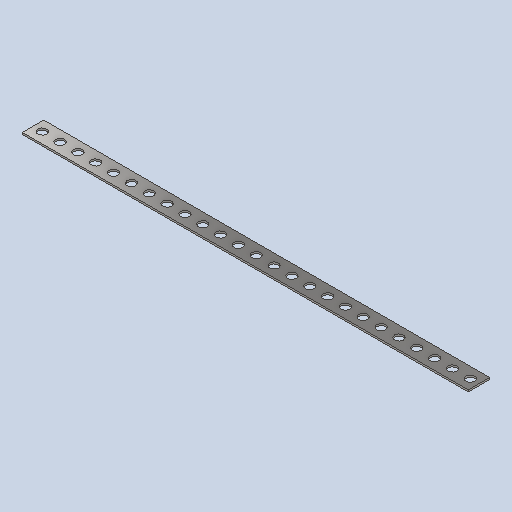
# Autodesk Inventor part: aste
Saved by Autodesk Inventor 2023 (Build 270158000, 158)
## iProperties
Created: 2023-08-07
Part Number: aste
Material: Aço, carbono
Document SubType Name: Modeling
Designer: azeve
Density: 7.85 g/cm^3
Appearance: Semipolido
Author: azeve
Autodesk Inventor part; units mm, degrees
ref_plane "YZ Plane" through (0, 0, 0) normal (1, 0, 0) x (0, 1, 0)
ref_plane "XZ Plane" through (0, 0, 0) normal (0, 1, 0) x (-1, 0, 0)
ref_plane "XY Plane" through (0, 0, 0) normal (0, 0, 1) x (1, 0, 0)
sketch "Esboço1" plane through (0, 0, 0) normal (0, 1, 0) x (-1, 0, 0)
  line L0 (0, 0) -> (250, 0)
  line L1 (250, 0) -> (250, 12)
  line L2 (250, 12) -> (0, 12)
  line L3 (0, 12) -> (0, 0)
  circle A0 centre (4.8421, 6) radius 2.5
  circle A1 centre (14.8421, 6) radius 2.5
  circle A2 centre (24.8421, 6) radius 2.5
  circle A3 centre (34.8421, 6) radius 2.5
  circle A4 centre (44.8421, 6) radius 2.5
  circle A5 centre (54.8421, 6) radius 2.5
  circle A6 centre (64.8421, 6) radius 2.5
  circle A7 centre (74.8421, 6) radius 2.5
  circle A8 centre (84.8421, 6) radius 2.5
  circle A9 centre (94.8421, 6) radius 2.5
  circle A10 centre (104.8421, 6) radius 2.5
  circle A11 centre (114.8421, 6) radius 2.5
  circle A12 centre (124.8421, 6) radius 2.5
  circle A13 centre (134.8421, 6) radius 2.5
  circle A14 centre (144.8421, 6) radius 2.5
  circle A15 centre (154.8421, 6) radius 2.5
  circle A16 centre (164.8421, 6) radius 2.5
  circle A17 centre (174.8421, 6) radius 2.5
  circle A18 centre (184.8421, 6) radius 2.5
  circle A19 centre (194.8421, 6) radius 2.5
  circle A20 centre (204.8421, 6) radius 2.5
  circle A21 centre (214.8421, 6) radius 2.5
  circle A22 centre (224.8421, 6) radius 2.5
  circle A23 centre (234.8421, 6) radius 2.5
  circle A24 centre (244.8421, 6) radius 2.5
  dimension "d0" = 250
  dimension "d1" = 12
  dimension "d2" = 5
  dimension "d8" = 10
  constraints: 25 centre point, 8 end point, 2 horizontal, 2 parallel, 1 perpendicular, 48 other
  measures "d0" distance of L2.end L1.end
  measures "d1" distance of L1.end L0.end
  measures "d2" diameter of A0
  measures "d8" distance of A0.centre A1.centre
extrude "Extrusão1" add sketch "Esboço1" along normal blind 1
